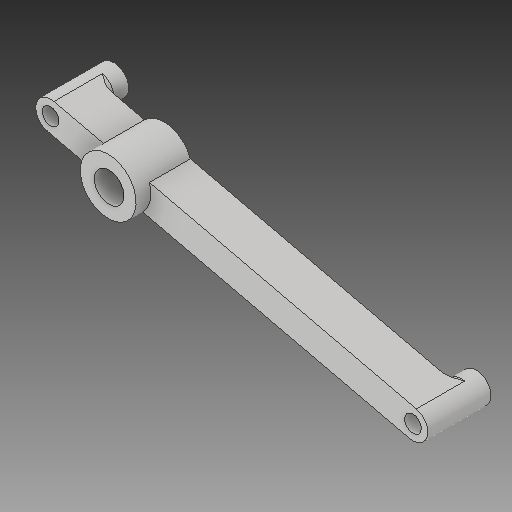
# Autodesk Inventor part: MassiveBone0
Saved by Autodesk Inventor 2017 (Build 210142000, 142)
## iProperties
Created: 2020-09-06
Part Number: MassiveBone0
Material: Generic
Document SubType Name: Modeling
Designer: agustin
Density: 1 g/cm^3
Appearance: Default
Author: agustin
Autodesk Inventor part; units mm, degrees
ref_plane "YZ Plane" through (0, 0, 0) normal (1, 0, 0) x (0, 1, 0)
ref_plane "XZ Plane" through (0, 0, 0) normal (0, 1, 0) x (-1, 0, 0)
ref_plane "XY Plane" through (0, 0, 0) normal (0, 0, 1) x (1, 0, 0)
sketch "Sketch1" plane through (0, 0, 0) normal (0, 0, 1) x (1, 0, 0)
  circle A0 centre (-0.795945, -40.492161) radius 2.25
  circle A1 centre (18.927108, -45.141259) radius 4
  circle A2 centre (96.560575, -63.333087) radius 2.25
  line L0 (-0.795945, -40.492161) -> (96.560575, -63.333087) construction
  arc A3 (0.117692, -36.5979) -> (-1.709582, -44.386422) centre (-0.795945, -40.492161) ccw
  arc A4 (95.646938, -67.227348) -> (97.474213, -59.438826) centre (96.560575, -63.333087) ccw
  arc A5 (11.352456, -46.680557) -> (24.513602, -49.768309) centre (18.675359, -45.060346) ccw
  line L1 (-1.709582, -44.386422) -> (11.585143, -47.505513)
  line L2 (23.938301, -50.403702) -> (95.646938, -67.227348)
  line L3 (97.474213, -59.438826) -> (25.765575, -42.61518)
  line L4 (13.412417, -39.716991) -> (0.117692, -36.5979)
  arc A6 (11.585143, -47.505513) -> (23.938301, -50.403702) centre (18.675359, -45.060346) ccw
  arc A7 (25.765575, -42.61518) -> (13.412417, -39.716991) centre (18.675359, -45.060346) ccw
  point P0 (0, 0)
  point P1 (47.882315, -51.912624)
  dimension "d0" = 8
  constraints: 12 end point, 8 point on circle, 8 tangent, 4 centre point, 4 parallel, 1 coincident, 1 midpoint
  measures "d0" diameter of A4
extrude "Extrusion1" add sketch "Sketch1" along normal blind 9
sketch "Sketch2" plane through (0, 0, 0) normal (0, 0, -1) x (-1, 0, 0)
  circle A0 centre (0.795945, -40.492161) radius 2.25
  circle A1 centre (-96.560575, -63.333087) radius 2.25
  circle A2 centre (-96.560575, -63.333087) radius 4
  circle A3 centre (0.795945, -40.492161) radius 4
  point P0 (0, 0)
  dimension "d3" = 8
  constraints: 2 centre point, 2 coincident
  measures "d3" diameter of A3
extrude "Extrusion2" add sketch "Sketch2" along normal blind 12
sketch "Sketch3" plane through (0, 0, 0) normal (0, 0, -1) x (-1, 0, 0)
  circle A0 centre (-18.927108, -45.141259) radius 4
  arc A1 (-95.646938, -67.227348) -> (-97.474213, -59.438826) centre (-96.560575, -63.333087) ccw
  line L0 (-95.646938, -67.227348) -> (-23.938301, -50.403702)
  arc A2 (-23.938301, -50.403702) -> (-11.585143, -47.505513) centre (-18.675359, -45.060346) ccw
  line L1 (-11.585143, -47.505513) -> (1.709582, -44.386422)
  arc A3 (-0.117692, -36.5979) -> (1.709582, -44.386422) centre (0.795945, -40.492161) ccw
  line L2 (-0.117692, -36.5979) -> (-13.412417, -39.716991)
  arc A4 (-13.412417, -39.716991) -> (-25.765575, -42.61518) centre (-18.675359, -45.060346) ccw
  line L3 (-25.765575, -42.61518) -> (-97.474213, -59.438826)
  point P0 (0, 0)
extrude "Extrusion3" add sketch "Sketch3" along normal blind 6
fillet "Fillet1" radius 2 3 edges at (3.0983, -41.4058, -6) (93.4257, -65.8176, -6) (94.0761, -60.1982, -6)
sketch "Sketch4" plane through (0, 0, 9) normal (0, 0, 1) x (1, 0, 0)
  arc A0 (11.585143, -47.505513) -> (23.938301, -50.403702) centre (18.675359, -45.060346) ccw
  circle A1 centre (18.927108, -45.141259) radius 4
  circle A2 centre (18.927108, -45.141259) radius 4
  circle A3 centre (96.560575, -63.333087) radius 2.25
  circle A4 centre (-0.795945, -40.492161) radius 2.25
  arc A5 (0.117692, -36.5979) -> (-1.709582, -44.386422) centre (-0.795945, -40.492161) ccw
  line L0 (-1.709582, -44.386422) -> (11.585143, -47.505513)
  arc A6 (11.585143, -47.505513) -> (23.938301, -50.403702) centre (18.675359, -45.060346) ccw
  line L1 (23.938301, -50.403702) -> (95.646938, -67.227348)
  arc A7 (95.646938, -67.227348) -> (97.474213, -59.438826) centre (96.560575, -63.333087) ccw
  line L2 (97.474213, -59.438826) -> (25.765575, -42.61518)
  arc A8 (25.765575, -42.61518) -> (13.412417, -39.716991) centre (18.675359, -45.060346) ccw
  line L3 (13.412417, -39.716991) -> (0.117692, -36.5979)
  circle A9 centre (18.675359, -45.060346) radius 7.5
  point P0 (0, 0)
  constraints: 1 coincident, 3 other
extrude "Extrusion4" cut sketch "Sketch4" against normal blind 4 contours L0 A5 L3 A9 | A9 L2 A7 L1
scale "Scale1" factors (0.5, 0.5, 0.5) then translate (28.807831, -29.152393, -3) bodies 1
body "Solid1"
